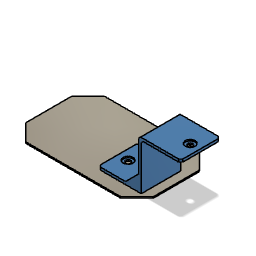
project012 v1 (Autodesk Fusion 360 design; units mm, degrees)
Autodesk Fusion 360 part; units mm, degrees
sketch "Sketch1" plane through (0, 0, 0) normal (0, 0, 1) x (1, 0, 0)
  line L0 (0, 0) -> (-65, 0)
  line L1 (0, 0) -> (0, 70)
  line L2 (0, 70) -> (60, 70)
  line L3 (-65, 0) -> (-65, 4)
  line L4 (-65, 4) -> (-4, 4)
  line L5 (-4, 4) -> (-4, 74)
  line L6 (-4, 74) -> (60, 74)
  line L7 (60, 74) -> (60, 70)
  dimension "d1" = 65
  dimension "d2" = 70
  dimension "d3" = 60
  dimension "d4" = 4
  dimension "d5" = 4
  dimension "d6" = 64
  dimension "d7" = 4
  constraint coincident L0.start L1.start
  constraint horizontal L0
  constraint perpendicular L0 L1
  constraint perpendicular L1 L2
  constraint perpendicular L0 L3
  constraint perpendicular L3 L4
  constraint perpendicular L4 L5
  constraint perpendicular L3 L6
  constraint perpendicular L2 L7
  measures "d1" distance of L0.start L0.end
  measures "d2" distance of L0.start L1.end
  measures "d3" distance of L1.end L2.end
  measures "d4" distance of L0.end L3.end
  measures "d5" distance of L1 L5
  measures "d6" distance of L5.end L6.end
  measures "d7" distance of L2 L6
extrude "Extrude1" add sketch "Sketch1" against normal blind 60 makes body 1
sketch "Sketch2" plane through (0, 74, 0) normal (0, 1, 0) x (-1, 0, 0)
  line L0 (4, 0) -> (-60, 0)
  line L1 (-60, 0) -> (-60, -60)
  line L2 (-60, -60) -> (4, -60)
  line L3 (4, -60) -> (4, 0)
  line L4 (-45, -68.4051) -> (-45, 9.8256) construction
  line L5 (-35, -30) -> (-85, -30) construction
  circle A0 centre (-45, -29.2898) radius 7.5
  dimension "d10" = 15
  dimension "d11" = 15
  constraint vertical L4
  constraint perpendicular L4 L5
  constraint midpoint L1 L5
  constraint midpoint L4 A0.centre
  measures "d10" distance of L1 L4
  measures "d11" diameter of A0
extrude "Extrude2" cut sketch "Sketch2" against normal blind 2 contours A0 bodies 1
sketch "Sketch3" plane through (0, 74, 0) normal (0, 1, 0) x (-1, 0, 0)
  circle A0 centre (-45, -29.2898) radius 7.5
  line L0 (4, 0) -> (-60, 0)
  line L1 (-60, 0) -> (-60, -60)
  line L2 (-60, -60) -> (4, -60)
  line L3 (4, -60) -> (4, 0)
  circle A1 centre (-45, -29.2898) radius 3.9443
  constraint concentric A0 A1
extrude "Extrude3" cut sketch "Sketch3" against normal blind 4 contours A1 bodies 1
sketch "Sketch4" plane through (0, 4, 0) normal (0, 1, 0) x (-1, 0, 0)
  line L0 (65, 0) -> (4, 0)
  line L1 (4, 0) -> (4, -60)
  line L2 (4, -60) -> (65, -60)
  line L3 (65, -60) -> (65, 0)
  line L4 (50, -66.7839) -> (50, -0.7237) construction
  line L5 (87.1984, -30) -> (42.8016, -30) construction
  circle A0 centre (50, -30) radius 7.5
  circle A1 centre (50, -30) radius 4
  dimension "d16" = 15
  dimension "d17" = 15
  constraint vertical L4
  constraint horizontal L5
  constraint midpoint L3 L5
  constraint coincident L5 A0.centre
  constraint concentric A0 A1
  measures "d16" distance of L3 L4
  measures "d17" diameter of A0
extrude "Extrude4" cut sketch "Sketch4" against normal blind 2 contours A0 bodies 1
extrude "Extrude5" cut 1 faces at (-49.7543, 4, -29.3803) along direction (0, -1, 0) blind 4 on bodies 1 bodies 1
chamfer "Chamfer1" distance 3 angle 45 1 edges at (-4, 74, -30) on bodies 1
chamfer "Chamfer2" distance 3 angle 45 1 edges at (0, 70, -30) on bodies 1
chamfer "Chamfer3" distance 3 angle 45 1 edges at (60, 72, 0) on bodies 1
chamfer "Chamfer4" distance 3 angle 45 3 edges at (60, 72, -60) (-65, 2, -60) (-65, 2, 0) on bodies 1
sketch "Sketch5" plane through (0, 0, 0) normal (0, 0, 1) x (1, 0, 0)
  line L0 (-62, 4) -> (-62, 0)
  line L1 (-62, 0) -> (0, 0)
  line L2 (0, 0) -> (0, 67)
  line L3 (0, 67) -> (3, 70)
  line L4 (3, 70) -> (57, 70)
  line L5 (57, 70) -> (57, 74)
  line L6 (57, 74) -> (-1, 74)
  line L7 (-1, 74) -> (-4, 71)
  line L8 (-4, 71) -> (-4, 4)
  line L9 (-4, 4) -> (-62, 4)
  line L10 (-4, 24) -> (-24, 4)
  dimension "d26" = 20
  dimension "d27" = 20
  constraint coincident L8 L10.start
  constraint coincident L9 L10.end
  measures "d26" distance of L8.end L10.start
  measures "d27" distance of L8.end L10.end
extrude "Extrude6" add sketch "Sketch5" against normal blind 6 contours L8 L9 L10 bodies 1
sketch "Sketch6" plane through (0, 0, -60) normal (0, 0, -1) x (-1, 0, 0)
  line L0 (62, 0) -> (62, 4)
  line L1 (62, 4) -> (4, 4)
  line L2 (4, 4) -> (4, 71)
  line L3 (4, 71) -> (1, 74)
  line L4 (1, 74) -> (-57, 74)
  line L5 (-57, 74) -> (-57, 70)
  line L6 (-57, 70) -> (-3, 70)
  line L7 (-3, 70) -> (0, 67)
  line L8 (0, 67) -> (0, 0)
  line L9 (0, 0) -> (62, 0)
  line L10 (4, 24) -> (24, 4)
  dimension "d30" = 20
  dimension "d31" = 20
  constraint coincident L2 L10.start
  constraint coincident L1 L10.end
  measures "d30" distance of L1.end L10.start
  measures "d31" distance of L1.end L10.end
extrude "Extrude7" add sketch "Sketch6" against normal blind 6 contours L1 L2 L10 bodies 1
sketch "Sketch7" plane through (0, 0, 0) normal (0, 1, 0) x (1, 0, 0)
  line L0 (-54.3851, -27.0099) -> (89.7793, -27.0099)
  line L1 (114.7793, -52.0099) -> (114.7793, -121.7351)
  line L2 (89.7793, -146.7351) -> (-54.3851, -146.7351)
  line L3 (-79.3851, -121.7351) -> (-79.3851, -52.0099)
  line L4 (89.7793, -27.0099) -> (114.7793, -52.0099)
  line L5 (-79.3851, -121.7351) -> (-54.3851, -146.7351)
  line L6 (-79.3851, -52.0099) -> (-54.3851, -27.0099)
  line L7 (89.7793, -146.7351) -> (114.7793, -121.7351)
  point P0 (-79.3851, -27.0099)
  point P1 (114.7793, -27.0099)
  point P2 (114.7793, -146.7351)
  point P3 (-79.3851, -146.7351)
  dimension "d34" = 25
  dimension "d35" = 25
  dimension "d36" = 25
  dimension "d37" = 25
  dimension "d38" = 25
  dimension "d39" = 25
  dimension "d40" = 25
  dimension "d41" = 25
  constraint horizontal L0
  constraint vertical L1
  constraint horizontal L2
  constraint vertical L3
  constraint coincident P1 L0
  constraint coincident P1 L1
  constraint coincident P3 L3
  constraint coincident P3 L2
  constraint coincident P0 L3
  constraint coincident P0 L0
  constraint coincident P2 L2
  constraint coincident P2 L1
  measures "d34" distance of P1 L0.end
  measures "d35" distance of P1 L1.start
  measures "d36" distance of P3 L3.start
  measures "d37" distance of P3 L2.end
  measures "d38" distance of P0 L3.end
  measures "d39" distance of P0 L0.start
  measures "d40" distance of P2 L2.start
  measures "d41" distance of P2 L1.end
extrude "Extrude8" add sketch "Sketch7" against normal blind 2 separate body makes body 2
copy_body "Body->Comp1" bodies 1 removing the originals makes body 3 in component "Component"
copy_body "Body->Comp2" bodies 2 removing the originals makes body 4 in component "Component'"
component "Component" placed x (1, 0, 0) y (0, -1, 0) z (0, 0, -1) at (101.6809, -2, 46.5074)
component "Component'" placed x (1, 0, 0) y (0, 1, 0) z (0, 0, 1) at (0, 0, 0)
equation "d35 = d34"
equation "d37 = d36"
equation "d39 = d38"
equation "d41 = d40"
